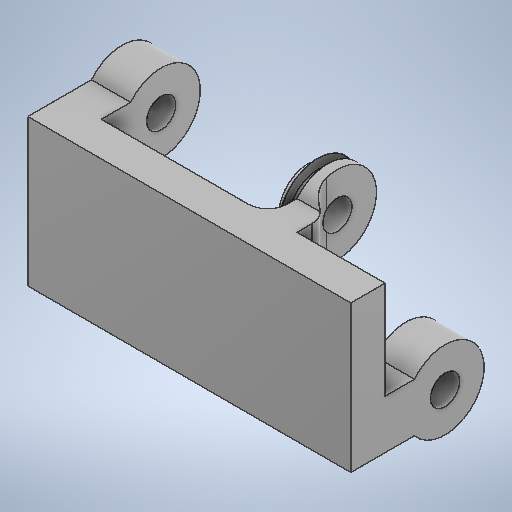
# Autodesk Inventor part: hausing_shaft_linkl
Saved by Autodesk Inventor 2025 (Build 290162000, 162)
## iProperties
Created: 2025-09-12
Part Number: hausing_shaft_linkl
Material: 一般
Document SubType Name: Modeling
Designer: sooo1
Density: 1 g/cm^3
Appearance: 滑らか - 標準の灰色
Author: sooo1
Autodesk Inventor part; units mm, degrees
sketch "スケッチ3" plane through (0, 0, 0) normal (1, 0, 0) x (0, 1, 0)
  line L0 (-12.6, 0) -> (12.6, 0) construction
  line L1 (0, -5.6) -> (0, 5.6) construction
  circle A0 centre (5, 0) radius 1.5
  circle A1 centre (-5, 0) radius 1.5
  circle A2 centre (5, 0) radius 4
  circle A3 centre (-5, 0) radius 4
  point P0 (0, 0)
  dimension "d13" = 5
  dimension "d14" = 5
  dimension "d15" = 3
  dimension "d16" = 8
  constraints: 4 centre point, 2 equal radius, 2 point on line
  measures "d13" distance from line of L1 A1.centre
  measures "d14" distance from line of L1 A0.centre
  measures "d15" diameter of A0
  measures "d16" diameter of A2
extrude "押し出し4" add sketch "スケッチ3" along normal mid plane 20 contours A2
ref_plane "作業平面2" through (-1, 0, 0) normal (1, 0, 0) x (0, 1, 0)
extrude "押し出し6" add sketch "スケッチ3" along normal blind 20 from surface at -1 contours A3
sketch "スケッチ4" plane through (0, 0, 0) normal (0, 0, 1) x (1, 0, 0)
  line L0 (-10, 9) -> (-10, 1) construction
  line L1 (10, 1) -> (10, 9) construction
  line L2 (-1, -1) -> (-1, -9) construction
  line L3 (19, -1) -> (19, -9) construction
  line L4 (-10, 1) -> (10, 1) construction
  line L5 (-8, 9) -> (8, 9)
  line L6 (8, 9) -> (8, 1)
  line L7 (8, 1) -> (-8, 1)
  line L8 (-8, 1) -> (-8, 9)
  line L9 (-8, 9) -> (8, 1) construction
  line L10 (8, 9) -> (-8, 1) construction
  line L11 (-10, 9) -> (10, 9) construction
  line L12 (0, 9) -> (0, 1) construction
  line L13 (-1, -1) -> (19, -1) construction
  line L14 (-1, -9) -> (19, -9) construction
  line L15 (1, -1) -> (17, -1)
  line L16 (17, -1) -> (17, -9)
  line L17 (17, -9) -> (1, -9)
  line L18 (1, -9) -> (1, -1)
  line L19 (1, -1) -> (17, -9) construction
  line L20 (17, -1) -> (1, -9) construction
  line L21 (9, -1) -> (9, -9) construction
  point P0 (0, 0)
  point P1 (0, 5)
  point P2 (9, -5)
  dimension "d24" = 16
  dimension "d25" = 16
  constraints: 28 end point, 10 midpoint, 4 parallel, 3 perpendicular, 2 collinear, 2 horizontal, 2 point on line
  measures "d24" distance of L5.start L5.end
  measures "d25" distance of L15.start L15.end
extrude "押し出し7" cut sketch "スケッチ4" along normal through all both and the other way through all
sketch "スケッチ5" plane through (0, 0, 0) normal (1, 0, 0) x (0, 1, 0)
  circle A0 centre (5, 0) radius 4 projected
  circle A1 centre (5, 0) radius 1.5 projected
  circle A2 centre (5, 0) radius 1.5 projected
  circle A3 centre (5, 0) radius 4 projected
  circle A4 centre (5, 0) radius 1.5 projected
  circle A5 centre (5, 0) radius 4 projected
  circle A6 centre (5, 0) radius 1.5 projected
  circle A7 centre (5, 0) radius 4 projected
  circle A8 centre (-5, 0) radius 4 projected
  circle A9 centre (-5, 0) radius 1.5 projected
  circle A10 centre (-5, 0) radius 4 projected
  circle A11 centre (-5, 0) radius 1.5 projected
  circle A12 centre (-5, 0) radius 4 projected
  circle A13 centre (-5, 0) radius 1.5 projected
  circle A14 centre (-5, 0) radius 1.5 projected
  circle A15 centre (-5, 0) radius 4 projected
  circle A16 centre (5, 0) radius 4 projected
  circle A17 centre (5, 0) radius 1.5 projected
  circle A18 centre (5, 0) radius 4 projected
  circle A19 centre (5, 0) radius 4 projected
  circle A20 centre (5, 0) radius 1.5 projected
  circle A21 centre (5, 0) radius 1.5 projected
  circle A22 centre (5, 0) radius 4 projected
  circle A23 centre (5, 0) radius 1.5 projected
  circle A24 centre (5, 0) radius 1.5 projected
  circle A25 centre (5, 0) radius 1.5 projected
  circle A26 centre (5, 0) radius 4 projected
  circle A27 centre (5, 0) radius 4 projected
  circle A28 centre (5, 0) radius 4 projected
  circle A29 centre (5, 0) radius 1.5 projected
  circle A30 centre (5, 0) radius 4 projected
  circle A31 centre (5, 0) radius 1.5 projected
  circle A32 centre (-5, 0) radius 4 projected
  circle A33 centre (-5, 0) radius 1.5 projected
  circle A34 centre (-5, 0) radius 4 projected
  circle A35 centre (-5, 0) radius 4 projected
  circle A36 centre (-5, 0) radius 1.5 projected
  circle A37 centre (-5, 0) radius 1.5 projected
  circle A38 centre (-5, 0) radius 1.5 projected
  circle A39 centre (-5, 0) radius 4 projected
  circle A40 centre (-5, 0) radius 1.5 projected
  circle A41 centre (-5, 0) radius 4 projected
  circle A42 centre (-5, 0) radius 4 projected
  circle A43 centre (-5, 0) radius 4 projected
  circle A44 centre (-5, 0) radius 1.5 projected
  circle A45 centre (-5, 0) radius 1.5 projected
  circle A46 centre (-5, 0) radius 4 projected
  circle A47 centre (-5, 0) radius 1.5 projected
  line L0 (7.5, 3.1225) -> (7.5, 8.1225)
  line L1 (7.5, 8.1225) -> (2.5, 8.1225)
  line L2 (2.5, 8.1225) -> (2.5, 3.1225)
  line L3 (-2.5, 3.1225) -> (-2.5, 8.1225)
  line L4 (-2.5, 8.1225) -> (-7.5, 8.1225)
  line L5 (-7.5, 8.1225) -> (-7.5, 3.1225)
  line L6 (5, 0) -> (5, 8.1225) construction
  line L7 (-5, 0) -> (-5, 8.1225) construction
  line L8 (7.5, 6.1225) -> (2.5, 6.1225)
  line L9 (-2.5, 6.1225) -> (-7.5, 6.1225)
  line L10 (2.5, 8.1225) -> (-2.5, 8.1225)
  line L11 (2.5, 6.1225) -> (-2.5, 6.1225)
  point P0 (0, 0)
  dimension "d28" = 5
  dimension "d29" = 5
  dimension "d34" = 2
  constraints: 24 end point, 9 point on line, 4 perpendicular, 4 point on circle, 3 midpoint, 3 parallel, 2 vertical, 1 collinear, 1 horizontal
  measures "d28" distance of L0.start L0.end
  measures "d29" distance of L0.end L1.end
  measures "d34" distance between parallel lines of L1 L8
extrude "押し出し8" add sketch "スケッチ5" along normal mid plane 20 contours A0 L2 L8 L0 | L8 L2 L1 L0
extrude "押し出し9" add sketch "スケッチ5" along normal blind 20 from surface at -1 contours L9 L5 L4 L3 | L3 A8 L5 L9
extrude "押し出し10" cut sketch "スケッチ5" along normal mid plane 16 contours A0 L2 L8 L0
extrude "押し出し11" cut sketch "スケッチ5" along normal up to surface (16 mm away) from surface at 1 contours L3 A8 L5 L9
extrude "押し出し12" add sketch "スケッチ5" along normal up to surface (11 mm away) from surface at -1 contours L11 L3 L10 L2
sketch "スケッチ6" plane through (-10, 7.5, 8.1225) normal (0, 0, 1) x (1, 0, 0)
  line L0 (9, -5) -> (0, -5) projected
  line L1 (9, -15) -> (9, -5) projected
  line L2 (20, 0) -> (20, -10) projected
  line L3 (20, -10) -> (29, -10) projected
  line L4 (2, -5) -> (9, -5) projected
  line L5 (0, -5) -> (1, -5)
  line L6 (9, -13) -> (9, -15)
  arc A0 (9, -13) -> (1, -5) centre (1, -13) ccw
  line L7 (20, 0) -> (20, -2)
  line L8 (28, -10) -> (29, -10)
  arc A1 (20, -2) -> (28, -10) centre (28, -2) ccw
  line L9 (0, -5) -> (0, -15)
  line L10 (0, -15) -> (9, -15)
  line L11 (20, 0) -> (29, 0)
  line L12 (29, 0) -> (29, -10)
  point P0 (10, -7.5)
  point P1 (1, -5)
  dimension "d41" = 8
  dimension "d42" = 8
  constraints: 16 end point, 4 perpendicular, 4 point on circle, 4 point on line, 4 tangent, 2 centre point, 2 collinear, 1 horizontal, 1 vertical
  measures "d41" radius of A0
  measures "d42" radius of A1
extrude "押し出し14" add sketch "スケッチ5" against normal blind 1 from surface at 8 contours A0
extrude "押し出し15" add sketch "スケッチ5" along normal blind 1 from surface at 1 contours A8
ref_plane "作業平面3" through (8.5, 5, 0) normal (-1, 0, 0) x (0, 0, 1)
ref_plane "作業平面4" through (0.5, -5, 0) normal (1, 0, 0) x (0, 0, -1)
sketch "スケッチ7" plane through (8.5, 5, 0) normal (-1, 0, 0) x (0, 0, 1)
  circle A0 centre (0, 0) radius 4 projected
  arc A1 (3.1225, -2.5) -> (3.1225, 2.5) centre (0, 0) ccw projected
  arc A2 (3.1225, 2.5) -> (3.1225, -2.5) centre (0, 0) ccw projected
  circle A3 centre (0, 0) radius 1.5 projected
  circle A4 centre (0, 0) radius 3
  arc A5 (3.1225, -2.5) -> (3.1225, 2.5) centre (0, 0) ccw projected
  line L0 (6.1225, -2.5) -> (3.1225, -2.5) projected
  line L1 (6.1225, 2.5) -> (6.1225, -2.5) projected
  line L2 (3.1225, 2.5) -> (6.1225, 2.5) projected
  point P0 (0, -5)
  point P1 (3.1225, 2.5)
  dimension "d49" = 1
  constraints: 1 centre point
  measures "d49" radial gap between concentric circles of A0 A4
extrude "押し出し16" cut sketch "スケッチ7" along normal mid plane 1 contours A0 | A0 L2 L1 L0
sketch "スケッチ8" plane through (0.5, -5, 0) normal (1, 0, 0) x (0, 0, -1)
  circle A0 centre (0, 0) radius 4 projected
  arc A1 (-3.1225, 2.5) -> (-3.1225, -2.5) centre (0, 0) ccw projected
  arc A2 (-3.1225, -2.5) -> (-3.1225, 2.5) centre (0, 0) ccw projected
  circle A3 centre (0, 0) radius 1.5 projected
  arc A4 (-3.1225, 2.5) -> (-3.1225, -2.5) centre (0, 0) ccw projected
  line L0 (-6.1225, 2.5) -> (-3.1225, 2.5) projected
  line L1 (-6.1225, 2.5) -> (-6.1225, -2.5) projected
  line L2 (-3.1225, -2.5) -> (-6.1225, -2.5) projected
  circle A5 centre (0, 0) radius 3
  point P0 (0, 5)
  point P1 (-3.1225, 2.5)
  point P2 (-3.1225, -2.5)
  dimension "d52" = 1
  constraints: 1 centre point
  measures "d52" radial gap between concentric circles of A5 A0
extrude "押し出し17" cut sketch "スケッチ8" along normal mid plane 1 contours A0 | A0 L2 L1 L0
fillet "フィレット1" radius 2 2 edges at (9, 5, 6.1225) (0, -5, 6.1225)
chamfer "面取り1" distance 1 angle 45 2 edges at (7, 1, 0) (2, -9, 0)
extrude "押し出し21" add sketch "スケッチ6" against normal up to surface (2 mm away) from surface at 0
sketch "スケッチ11" plane through (19, -5, 0) normal (1, 0, 0) x (0, 0, -1)
  circle A0 centre (0, 0) radius 1.5 projected
  arc A1 (-3.1225, -2.5) -> (-3.1225, 2.5) centre (0, 0) ccw projected
  line L0 (-6.1225, 2.5) -> (-3.1225, 2.5) projected
  line L1 (-6.1225, 12.5) -> (-6.1225, 2.5) projected
  line L2 (-8.1225, 12.5) -> (-6.1225, 12.5) projected
  line L3 (-8.1225, -2.5) -> (-8.1225, 12.5) projected
  line L4 (-3.1225, -2.5) -> (-8.1225, -2.5) projected
  circle A2 centre (0, 10) radius 1.5 projected
  line L5 (-6.1225, 12.5) -> (-6.1225, 7.5) projected
  line L6 (-6.1225, 7.5) -> (-3.1225, 7.5) projected
  arc A3 (-3.1225, 7.5) -> (-3.1225, 12.5) centre (0, 10) ccw projected
  line L7 (-3.1225, 12.5) -> (-6.1225, 12.5) projected
  line L8 (-3.1225, 12.5) -> (-3.1225, 7.5)
  line L9 (-6.1225, -2.5) -> (-6.1225, 2.5) projected
  line L10 (-6.1225, 2.5) -> (-6.1225, -2.5)
  line L11 (-3.1225, 2.5) -> (-3.1225, -2.5)
  line L12 (-6.1225, 2.5) -> (-8.1225, 2.5)
  line L13 (-6.1225, -2.5) -> (-6.1225, 7.5) projected
  line L14 (-6.1225, 7.5) -> (-8.1225, 7.5)
  point P0 (0, 5)
  point P1 (-6.1225, 12.5)
  point P2 (-6.1225, 7.5)
  point P3 (-6.1225, 12.5)
  constraints: 10 end point, 2 perpendicular, 2 point on line, 2 vertical, 1 parallel
extrude "押し出し22" add sketch "スケッチ11" along normal blind 2 contours L11 A1 | L4 L9 L0 L11 | L4 L3 L12 L9 | L12 L3 L14 L1 | L14 L3 L2 L1
extrude "押し出し23" add sketch "スケッチ11" along normal blind 2 from surface at -9 contours L1 L7 L8 L6
extrude "押し出し24" add sketch "スケッチ11" against normal blind 2 from surface at -29 contours L4 L3 L12 L9 | L12 L3 L14 L1 | L14 L3 L2 L1 | L1 L7 L8 L6 | L8 A3
extrude "押し出し25" add sketch "スケッチ11" against normal blind 2 from surface at -20 contours L4 L9 L0 L11
fillet "フィレット2" radius 2 4 edges at (12, 5, 3.1225) (10, 5, 3.1225) (-1, -5, 3.1225) (-3, -5, 3.1225)
sketch "スケッチ12" plane through (21, -7.5, 8.1225) normal (0, 0, 1) x (1, 0, 0)
  line L0 (-33, 0) -> (0, 0) projected
  line L1 (0, 15) -> (0, 0) projected
  line L2 (-33, 15) -> (0, 15) projected
  line L3 (-33, 0) -> (-33, 15) projected
  point P0 (-21, 7.5)
extrude "押し出し26" add sketch "スケッチ12" along normal blind 1.5
